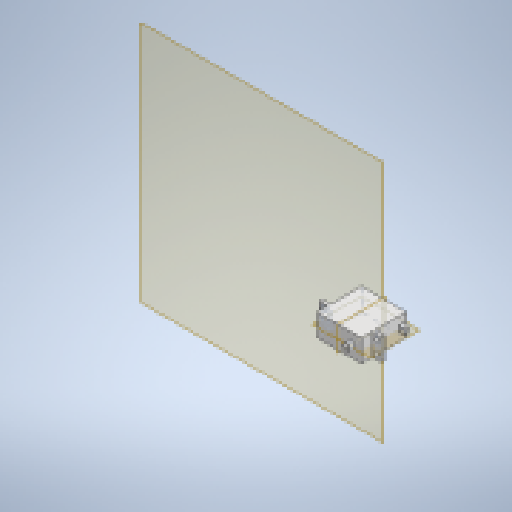
# Autodesk Inventor part: Servomotor
Saved by Autodesk Inventor 2024 (Build 280153000, 153)
## iProperties
Created: 2024-07-18
Part Number: Servomotor
Material: Genérico
Document SubType Name: Modeling
Designer: sergi
Density: 1 g/cm^3
Appearance: Valor por defecto
Author: sergi
Autodesk Inventor part; units mm, degrees
ref_plane "YZ Plane" through (0, 0, 0) normal (1, 0, 0) x (0, 1, 0)
ref_plane "XZ Plane" through (0, 0, 0) normal (0, 1, 0) x (-1, 0, 0)
ref_plane "XY Plane" through (0, 0, 0) normal (0, 0, 1) x (1, 0, 0)
ref_plane "Plano de trabajo1" through (-110.1, 7.287, 0) normal (0, 0, 1) x (0, 1, 0)
sketch "Boceto1" plane through (-110.1, 7.287, 0) normal (0, 0, 1) x (0, 1, 0)
  line L0 (-17.387, -89.9) -> (2.813, -89.9)
  line L1 (2.813, -89.9) -> (2.813, -130.3)
  line L2 (2.813, -130.3) -> (-17.387, -130.3)
  line L3 (-17.387, -130.3) -> (-17.387, -89.9)
  line L4 (-17.387, -89.9) -> (2.813, -130.3) construction
  line L5 (2.813, -89.9) -> (-17.387, -130.3) construction
  point P0 (-7.287, -110.1)
  dimension "d0" = 20.2
  dimension "d1" = 40.4
  constraints: 12 end point, 2 midpoint, 2 parallel, 1 horizontal, 1 perpendicular
  measures "d0" distance of L1.end L2.end
  measures "d1" distance of L0.end L1.end
extrude "Extrusión1" add sketch "Boceto1" along normal blind 40.4
sketch "Boceto2" plane through (20.2, -10.1, 0) normal (1, 0, 0) x (0, 1, 0)
  line L0 (0, 0) -> (20.2, 0) projected
  line L1 (20.2, 0) -> (20.2, 40.4) projected
  line L2 (0, 40.4) -> (20.2, 40.4) projected
  line L3 (0, 0) -> (0, 40.4) projected
  line L4 (20.2, 0) -> (0, 0) projected
  line L5 (0, 0) -> (0, 27.7)
  line L6 (0, 27.7) -> (20.2, 27.7)
  line L7 (0, 27.7) -> (20.2, 27.7)
  line L8 (20.2, 27.7) -> (20.2, 30.45)
  line L9 (20.2, 30.45) -> (0, 30.45)
  line L10 (0, 30.45) -> (0, 27.7)
  point P0 (10.1, 0)
  dimension "d4" = 27.7
  dimension "d5" = 2.75
  constraints: 12 end point, 3 point on line, 2 parallel, 2 perpendicular, 1 horizontal
  measures "d4" distance of L0.start L5.end
  measures "d5" distance of L8.end L7.end
extrude "Extrusión2" add sketch "Boceto2" along normal blind 8 contours L3 L9 L1 L6
sketch "Boceto3" plane through (20.2, -10.1, 30.45) normal (0, 0, 1) x (0, 1, 0)
  line L0 (0, -8) -> (20.2, -8) projected
  line L1 (0, -8) -> (0, -2.25)
  line L2 (0, 0) -> (0, -8) projected
  line L3 (0, -2.25) -> (20.2, -2.25)
  line L4 (0, 0) -> (20.2, 0) projected
  line L5 (0, 0) -> (0, -8) projected
  line L6 (20.2, -8) -> (0, -8) projected
  line L7 (20.2, 0) -> (20.2, -8) projected
  line L8 (0, -2.25) -> (2.8, -2.25)
  line L9 (0, -2.25) -> (2.8, -2.25) construction
  line L10 (2.8, -2.25) -> (2.8, -8)
  line L11 (20.2, -8) -> (0, -8) projected
  circle A0 centre (5, -4.45) radius 2.2
  point P0 (10.1, 20.2)
  dimension "d8" = 5.75
  dimension "d9" = 2.8
  dimension "d10" = 0
  dimension "d11" = 90
  dimension "d12" = 4.4
  constraints: 10 end point, 3 point on line, 2 collinear, 2 tangent, 1 centre point, 1 horizontal, 1 perpendicular
  measures "d8" distance of L0.start L1.end
  measures "d9" distance of L1.end L8.end
  measures "d10" distance between parallel lines of L8 L9
  measures "d11" angle of L8 L10
  measures "d12" diameter of A0
hole "Agujero1" at (24.65, -5.1, 30.45) direction (0, 0, -1) diameter 4.4 end through all
ref_plane "Plano de trabajo2" through (20.2, 0, 0) normal (0, 1, 0) x (0, 0, -1)
mirror "Simetría1" about plane through (20.2, 0, 0) normal (0, 1, 0) of "Agujero1"
ref_plane "Plano de trabajo3" through (0, -10.1, 0) normal (1, 0, 0) x (0, 1, 0)
mirror "Simetría2" about plane through (0, -10.1, 0) normal (1, 0, 0) of "Extrusión2", "Agujero1", "Simetría1"
sketch "Boceto4" plane through (-110.1, 7.287, 40.4) normal (0, 0, 1) x (0, 1, 0)
  line L0 (-17.387, -130.3) -> (2.813, -130.3) projected
  line L1 (2.813, -130.3) -> (2.813, -89.9) projected
  line L2 (2.813, -89.9) -> (-17.387, -89.9) projected
  line L3 (-17.387, -89.9) -> (-17.387, -130.3) projected
  line L4 (-17.387, -130.3) -> (2.813, -130.3) projected
  line L5 (-7.287, -130.3) -> (-7.287, -123.6)
  line L6 (-7.287, -123.6) -> (-7.287, -117.6)
  circle A0 centre (-7.287, -120.6) radius 3
  point P0 (-7.287, -110.1)
  dimension "d20" = 6.7
  dimension "d21" = 6
  constraints: 4 end point, 2 midpoint, 1 point on line, 1 vertical, 1 vertical alignment, 2 other
  measures "d20" distance of L5.start L5.end
  measures "d21" distance of L5.end L6.end
extrude "Extrusión3" add sketch "Boceto4" along normal blind 4 contours A0 L6 | L6 A0
sketch "Boceto5" plane through (10.5, 0, 44.4) normal (0, 0, 1) x (1, 0, 0)
  circle A0 centre (0, 0) radius 3 projected
  point P0 (-10.5, 0)
  constraints: 1 coincident
hole "Agujero2" at (10.5, 0, 44.4) direction (0, 0, -1) diameter 4.4 depth 6.5
sketch "Boceto6" plane through (20.2, -10.1, 0) normal (1, 0, 0) x (0, 1, 0)
  line L0 (20.2, 0) -> (20.2, 27.7) projected
  line L1 (0, 0) -> (20.2, 0)
  line L2 (20.2, 0) -> (20.2, 6.45)
  line L3 (20.2, 6.45) -> (0, 6.45)
  line L4 (0, 6.45) -> (0, 0)
  line L5 (0, 0) -> (20, 0)
  line L6 (20, 0) -> (20, 2.75)
  line L7 (20, 2.75) -> (0, 2.75)
  line L8 (0, 2.75) -> (0, 0)
  line L9 (0, 2.75) -> (7.5, 2.75)
  line L10 (7.5, 2.75) -> (7.5, 6.45)
  line L11 (20.2, 6.45) -> (12.7, 6.45)
  line L12 (7.5, 2.75) -> (12.7, 2.75)
  line L13 (12.7, 2.75) -> (12.7, 6.45)
  line L14 (12.7, 6.45) -> (7.5, 6.45)
  line L15 (7.5, 6.45) -> (7.5, 2.75)
  point P0 (10.1, 0)
  dimension "d31" = 6.45
  dimension "d32" = 2.75
  dimension "d33" = 7.5
  dimension "d34" = 7.5
  constraints: 30 end point, 6 parallel, 4 perpendicular, 4 point on line, 3 horizontal
  measures "d31" distance of L2.end L1.end
  measures "d32" distance of L6.end L5.end
  measures "d33" distance of L7.end L9.end
  measures "d34" distance of L2.end L11.end
extrude "Extrusión4" add sketch "Boceto6" along normal blind 5 contours L13 L7 L10 L3
